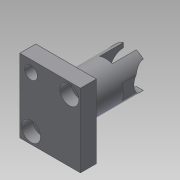
# Autodesk Inventor part: Фиксатор
Saved by Autodesk Inventor 2014 SP1 (Build 180222100, 222)
## iProperties
Created: 2014-04-11
Part Number: Фиксатор
Material: Типовые
Document SubType Name: Modeling
Designer: Украинцев
Mass: 28.6999 g
Surface Area: 89.0799 cm^2
Volume: 28.6999 cm^3
Density: 1 g/cm^3
Appearance: По умолчанию
Author: Украинцев
Autodesk Inventor part; units mm, degrees
ref_plane "YZ Plane" through (0, 0, 0) normal (1, 0, 0) x (0, 1, 0)
ref_plane "XZ Plane" through (0, 0, 0) normal (0, 1, 0) x (-1, 0, 0)
ref_plane "XY Plane" through (0, 0, 0) normal (0, 0, 1) x (1, 0, 0)
sketch "Эскиз1" plane through (0, 0, 0) normal (0, 0, 1) x (1, 0, 0)
  line L0 (-19, 10) -> (19, 10)
  line L1 (19, 10) -> (19, 0)
  line L2 (19, 0) -> (-19, 0)
  line L3 (-19, 0) -> (-19, 10)
  line L4 (12, 10) -> (12, 34)
  line L5 (12, 34) -> (11, 34)
  line L6 (11, 34) -> (11, 50)
  line L7 (11, 50) -> (4, 50)
  line L8 (4, 50) -> (4, 35)
  line L9 (4, 35) -> (0, 35)
  line L10 (0, 35) -> (0, 10)
  line L11 (12, 34) -> (12, 50)
  line L12 (12, 50) -> (11, 50)
  line L13 (4, 50) -> (-4, 50)
  line L14 (-4, 50) -> (-4, 35)
  line L15 (-4, 35) -> (0, 35)
  line L16 (-12, 34) -> (-11, 34)
  line L17 (-11, 34) -> (-11, 50)
  line L18 (-12, 34) -> (-12, 50)
  line L19 (-12, 50) -> (-11, 50)
  point P0 (0, 0)
  point P1 (0, 0)
  dimension "d0" = 38
  dimension "d1" = 50
  dimension "d2" = 40
  dimension "d3" = 16
  dimension "d4" = 15
  dimension "d5" = 22
  dimension "d6" = 4
  dimension "d7" = 24
  dimension "d13" = 8
  constraints: 40 end point, 9 parallel, 4 perpendicular, 4 symmetric about line, 2 midpoint, 1 coincident, 1 collinear, 1 horizontal, 1 point on line
  measures "d0" distance of L1.end L2.end
  measures "d1" distance between parallel lines of L7 L2
  measures "d2" distance between parallel lines of L0 L7
  measures "d3" distance between parallel lines of L5 L7
  measures "d4" distance between parallel lines of L9 L7
  measures "d5" diameter of L6 L10
  measures "d6" distance from line of L9.end L8
  measures "d7" diameter of L4 L10
  measures "d13" distance of L7.end L13.end
extrude "Выдавливание1" add sketch "Эскиз1" along normal mid plane 46 contours L0 L1 L2 L3
revolve "Вращение1" add sketch "Эскиз1" angle 360 about axis through (0, 35, 0) along (0, -1, 0) contours L10 L9 L8 L7 L6 L5 L4 L0 | L5 L6 L12 L11
extrude "Выдавливание2" cut sketch "Эскиз1" along normal through all both and the other way through all contours L15 L14 L13 L8 L9 | L5 L6 L12 L11 | L18 L19 L17 L16
sketch "Эскиз2" plane through (-11, 34, 4.7958) normal (-1, 0, 0) x (0, 0, 1)
  arc A0 (-13.2958, 16) -> (3.7042, 16) centre (-4.7958, 16) ccw
  line L0 (-13.2958, 16) -> (3.7042, 16)
  line L1 (6.5179, 16) -> (-16.1095, 16) projected
  point P0 (-4.7958, 16)
  dimension "d16" = 8.5
  constraints: 2 end point, 2 midpoint, 2 point on circle, 1 centre point, 1 coincident, 1 horizontal
  measures "d16" radius of A0
extrude "Выдавливание4" cut sketch "Эскиз2" against normal through all
sketch "Эскиз3" plane through (-19, 0, 23) normal (0, -1, 0) x (1, 0, 0)
  point P0 (19, -23)
  point P1 (7, -7)
  point P2 (7, -39)
  point P3 (31, -7)
  dimension "d19" = 12
  dimension "d21" = 16
  dimension "d22" = 32
  dimension "d30" = 24
  constraints: 1 horizontal alignment, 1 vertical alignment
  measures "d19" horizontal distance of point (7, -7) point (19, -23)
  measures "d21" vertical distance of point (7, -7) point (19, -23)
  measures "d22" distance of point (7, -39) point (7, -7)
  measures "d30" distance of point (31, -7) point (7, -7)
hole "Отверстие1" at (-12, 0, 16) direction (0, 1, 0) diameter 8 end through all
hole "Отверстие2" at (12, 0, 16) at (-12, 0, -16) direction (0, 1, 0) diameter 7 end through all counterbore diameter 12 counterbore depth 7
